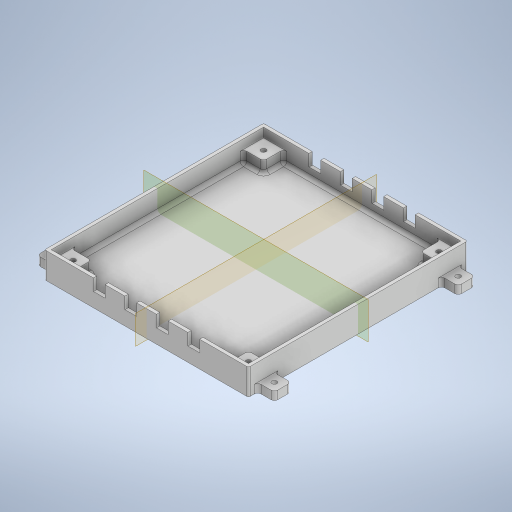
# Autodesk Inventor part: Case
Saved by Autodesk Inventor 2023.5 (Build 275446000, 446)
## iProperties
Created: 2025-10-09
Part Number: Case
Material: Generic
Document SubType Name: Modeling
Designer: Mikke
Density: 1 g/cm^3
Appearance: Default
Author: Mikke
Autodesk Inventor part; units mm, degrees
ref_plane "YZ Plane" through (0, 0, 0) normal (1, 0, 0) x (0, 1, 0)
ref_plane "XZ Plane" through (0, 0, 0) normal (0, 1, 0) x (-1, 0, 0)
ref_plane "XY Plane" through (0, 0, 0) normal (0, 0, 1) x (1, 0, 0)
sketch "Sketch1" plane through (0, 0, 0) normal (0, 1, 0) x (-1, 0, 0)
  line L0 (-61, 65.5) -> (61, 65.5)
  line L1 (61, 65.5) -> (61, -65.5)
  line L2 (61, -65.5) -> (-61, -65.5)
  line L3 (-61, -65.5) -> (-61, 65.5)
  line L4 (-61, 65.5) -> (61, -65.5) construction
  line L5 (61, 65.5) -> (-61, -65.5) construction
  point P0 (0, 0)
  dimension "d0" = 122
  dimension "d1" = 131
  constraints: 12 end point, 2 midpoint, 2 parallel, 1 horizontal, 1 perpendicular
  measures "d0" distance of L1.end L2.end
  measures "d1" distance of L0.end L1.end
extrude "Extrusion1" add sketch "Sketch1" along normal blind 3
sketch "Sketch2" plane through (0, 3, 0) normal (0, 1, 0) x (1, 0, 0)
  line L0 (59, -63.5) -> (-59, -63.5)
  line L1 (-59, -63.5) -> (-59, 63.5)
  line L2 (-59, 63.5) -> (59, 63.5)
  line L3 (59, 63.5) -> (59, -63.5)
  line L4 (59, -63.5) -> (-59, 63.5) construction
  line L5 (-59, -63.5) -> (59, 63.5) construction
  line L6 (-59, -63.5) -> (-53, -63.5)
  line L7 (-53, -63.5) -> (-53, -57.5)
  line L8 (-53, -57.5) -> (-59, -57.5)
  line L9 (-59, -57.5) -> (-59, -63.5)
  line L10 (-59, 63.5) -> (-53, 63.5)
  line L11 (-53, 63.5) -> (-53, 57.5)
  line L12 (-53, 57.5) -> (-59, 57.5)
  line L13 (-59, 57.5) -> (-59, 63.5)
  circle A0 centre (-53, -57.5) radius 1.5
  line L14 (-59, -63.5) -> (-47, -63.5)
  line L15 (-47, -63.5) -> (-47, -51.5)
  line L16 (-47, -51.5) -> (-59, -51.5)
  line L17 (-59, -51.5) -> (-59, -63.5)
  circle A1 centre (-53, 57.5) radius 1.5
  line L18 (-59, 63.5) -> (-47, 63.5)
  line L19 (-47, 63.5) -> (-47, 51.5)
  line L20 (-47, 51.5) -> (-59, 51.5)
  line L21 (-59, 51.5) -> (-59, 63.5)
  line L22 (59, 63.5) -> (53, 63.5)
  line L23 (53, 63.5) -> (53, 57.5)
  line L24 (53, 57.5) -> (59, 57.5)
  line L25 (59, 57.5) -> (59, 63.5)
  line L26 (59, 63.5) -> (47, 63.5)
  line L27 (47, 63.5) -> (47, 51.5)
  line L28 (47, 51.5) -> (59, 51.5)
  line L29 (59, 51.5) -> (59, 63.5)
  circle A2 centre (53, 57.5) radius 1.5
  line L30 (59, -63.5) -> (53, -63.5)
  line L31 (53, -63.5) -> (53, -57.5)
  line L32 (53, -57.5) -> (59, -57.5)
  line L33 (59, -57.5) -> (59, -63.5)
  line L34 (59, -63.5) -> (47, -63.5)
  line L35 (47, -63.5) -> (47, -51.5)
  line L36 (47, -51.5) -> (59, -51.5)
  line L37 (59, -51.5) -> (59, -63.5)
  circle A3 centre (53, -57.5) radius 1.5
  point P0 (0, 0)
  dimension "d4" = 118
  dimension "d5" = 127
  dimension "d6" = 6
  dimension "d7" = 6
  dimension "d8" = 6
  dimension "d9" = 6
  dimension "d11" = 3
  dimension "d12" = 12
  dimension "d13" = 12
  dimension "d14" = 3
  dimension "d15" = 12
  dimension "d16" = 12
  dimension "d17" = 6
  dimension "d18" = 6
  dimension "d19" = 12
  dimension "d20" = 12
  dimension "d21" = 3
  dimension "d22" = 6
  dimension "d23" = 6
  dimension "d24" = 12
  dimension "d25" = 12
  dimension "d26" = 3
  constraints: 76 end point, 18 parallel, 9 horizontal, 9 perpendicular, 4 centre point, 4 coincident, 2 midpoint
  measures "d4" distance of L1.end L2.end
  measures "d5" distance of L0.end L1.end
  measures "d6" distance of L8.end L7.end
  measures "d7" distance of L7.end L6.end
  measures "d8" distance of L11.end L12.end
  measures "d9" distance of L10.end L11.end
  measures "d11" diameter of A0
  measures "d12" distance of L16.end L15.end
  measures "d13" distance of L15.end L14.end
  measures "d14" diameter of A1
  measures "d15" distance of L19.end L20.end
  measures "d16" distance of L18.end L19.end
  measures "d17" distance of L24.end L23.end
  measures "d18" distance of L23.end L22.end
  measures "d19" distance of L28.end L27.end
  measures "d20" distance of L27.end L26.end
  measures "d21" diameter of A2
  measures "d22" distance of L31.end L32.end
  measures "d23" distance of L30.end L31.end
  measures "d24" distance of L35.end L36.end
  measures "d25" distance of L34.end L35.end
  measures "d26" diameter of A3
extrude "Extrusion2" add sketch "Sketch2" along normal blind 7 contours L0 L31 A3 L32 L3 | L0 L35 L36 L3 L32 A3 L31 | A3 L32 L31 | L31 L32 A3 | L0 L7 A0 L8 L1 L16 L15 | L28 L27 L2 L23 A2 L24 L3 | L0 L1 L8 A0 L7 | L24 A2 L23 L2 L3 | A0 L8 L7 | L7 L8 A0 | A2 L23 L24 | L24 L23 A2 | L1 L12 A1 L11 L2 L19 L20 | L1 L2 L11 A1 L12 | A1 L11 L12 | L12 L11 A1
sketch "Sketch3" plane through (0, 3, 0) normal (0, 1, 0) x (1, 0, 0)
  line L0 (-61, 65.5) -> (-61, -65.5) projected
  line L1 (61, 65.5) -> (-61, 65.5) projected
  line L2 (-61, -65.5) -> (61, -65.5)
  line L3 (61, -65.5) -> (61, 65.5)
  line L4 (61, 65.5) -> (-61, 65.5)
  line L5 (-61, 65.5) -> (-61, -65.5)
  line L6 (-59, -63.5) -> (-59, -51.5) projected
  line L7 (59, 63.5) -> (59, 51.5) projected
  line L8 (-59, -63.5) -> (59, -63.5)
  line L9 (59, -63.5) -> (59, 63.5)
  line L10 (59, 63.5) -> (-59, 63.5)
  line L11 (-59, 63.5) -> (-59, -63.5)
  point P0 (0, 0)
  constraints: 16 end point, 4 parallel, 2 horizontal, 2 perpendicular
extrude "Extrusion3" add sketch "Sketch3" along normal blind 12.5
sketch "Sketch5" plane through (47, 3, 63.5) normal (0, 0, -1) x (-1, 0, 0)
  line L0 (-12, 12.5) -> (106, 12.5) projected
  line L1 (0, 7) -> (94, 7)
  line L2 (94, 7) -> (94, 8.5)
  line L3 (94, 8.5) -> (0, 8.5)
  line L4 (0, 8.5) -> (0, 7)
  line L5 (47, 12.5) -> (47, 8.5)
  line L6 (47, 8.5) -> (0, 8.5)
  line L7 (47, 8.5) -> (94, 8.5)
  line L8 (47, 8.5) -> (18.642, 8.5)
  line L9 (47, 8.5) -> (37.575, 8.5)
  line L10 (47, 8.5) -> (56.425, 8.5)
  line L11 (56.425, 8.5) -> (75.283, 8.5)
  line L12 (37.575, 8.5) -> (18.717, 8.5)
  line L13 (18.717, 8.5) -> (18.717, 9)
  line L14 (37.575, 8.5) -> (37.575, 9)
  line L15 (56.425, 8.5) -> (56.425, 9)
  line L16 (75.283, 8.5) -> (75.283, 9)
  line L17 (71.783, 5.5) -> (78.783, 5.5)
  line L18 (78.783, 5.5) -> (78.783, 12.5)
  line L19 (78.783, 12.5) -> (71.783, 12.5)
  line L20 (71.783, 12.5) -> (71.783, 5.5)
  line L21 (71.783, 5.5) -> (78.783, 12.5) construction
  line L22 (78.783, 5.5) -> (71.783, 12.5) construction
  line L23 (52.925, 5.5) -> (59.925, 5.5)
  line L24 (59.925, 5.5) -> (59.925, 12.5)
  line L25 (59.925, 12.5) -> (52.925, 12.5)
  line L26 (52.925, 12.5) -> (52.925, 5.5)
  line L27 (52.925, 5.5) -> (59.925, 12.5) construction
  line L28 (59.925, 5.5) -> (52.925, 12.5) construction
  line L29 (34.075, 5.5) -> (41.075, 5.5)
  line L30 (41.075, 5.5) -> (41.075, 12.5)
  line L31 (41.075, 12.5) -> (34.075, 12.5)
  line L32 (34.075, 12.5) -> (34.075, 5.5)
  line L33 (34.075, 5.5) -> (41.075, 12.5) construction
  line L34 (41.075, 5.5) -> (34.075, 12.5) construction
  line L35 (15.217, 5.5) -> (22.217, 5.5)
  line L36 (22.217, 5.5) -> (22.217, 12.5)
  line L37 (22.217, 12.5) -> (15.217, 12.5)
  line L38 (15.217, 12.5) -> (15.217, 5.5)
  line L39 (15.217, 5.5) -> (22.217, 12.5) construction
  line L40 (22.217, 5.5) -> (15.217, 12.5) construction
  point P0 (47, -3)
  point P1 (47, -3)
  dimension "d31" = 1.5
  dimension "d33" = 9.425
  dimension "d34" = 9.425
  dimension "d35" = 18.858
  dimension "d36" = 18.858
  dimension "d37" = 0.5
  dimension "d38" = 0.5
  dimension "d39" = 0.5
  dimension "d40" = 0.5
  dimension "d41" = 7
  dimension "d42" = 7
  dimension "d43" = 7
  dimension "d44" = 7
  dimension "d45" = 7
  dimension "d46" = 7
  dimension "d47" = 7
  dimension "d48" = 7
  constraints: 80 end point, 10 midpoint, 9 equal length, 8 perpendicular, 5 horizontal, 5 point on line, 3 vertical, 1 coincident
  measures "d31" distance of L1.end L2.end
  measures "d33" distance of L5.end L9.end
  measures "d34" distance of L5.end L10.end
  measures "d35" distance of L10.end L11.end
  measures "d36" distance of L9.end L12.end
  measures "d37" distance of L12.end L13.end
  measures "d38" distance of L9.end L14.end
  measures "d39" distance of L10.end L15.end
  measures "d40" distance of L11.end L16.end
  measures "d41" distance of L19.end L18.end
  measures "d42" distance of L18.end L17.end
  measures "d43" distance of L25.end L24.end
  measures "d44" distance of L24.end L23.end
  measures "d45" distance of L31.end L30.end
  measures "d46" distance of L30.end L29.end
  measures "d47" distance of L37.end L36.end
  measures "d48" distance of L36.end L35.end
extrude "Extrusion4" cut sketch "Sketch5" against normal blind 3 contours L0 L36 L3 L38 | L3 L36 L1 L38 | L0 L30 L3 L32 | L1 L36 L35 L38 | L3 L30 L1 L32 | L1 L30 L29 L32 | L0 L24 L3 L26 | L3 L24 L1 L26 | L1 L24 L23 L26 | L0 L18 L3 L20 | L3 L18 L1 L20 | L1 L18 L17 L20
ref_plane "Work Plane1" through (47, 3, 0) normal (0, 0, -1) x (-1, 0, 0)
mirror "Mirror1" about plane through (47, 3, 0) normal (0, 0, -1) of "Extrusion4"
fillet "Fillet1" radius 2 24 edges at (-47, 3, 57.5) (0, 3, 63.5) (-53, 3, 51.5) (-47, 6.5, 51.5) (-47, 6.5, 63.5) (-59, 6.5, 51.5) (-59, 3, 0) (47, 3, 57.5) (47, 6.5, 51.5) (47, 6.5, 63.5) (53, 3, 51.5) (59, 3, 0) (59, 6.5, 51.5) (53, 3, -51.5) (59, 6.5, -51.5) (47, 6.5, -51.5) (47, 3, -57.5) (47, 6.5, -63.5) (0, 3, -63.5) (-59, 6.5, -51.5) (-53, 3, -51.5) (-47, 6.5, -51.5) (-47, 3, -57.5) (-47, 6.5, -63.5)
fillet "Fillet2" radius 1 4 edges at (-61, 7.75, -65.5) (61, 7.75, -65.5) (61, 7.75, 65.5) (-61, 7.75, 65.5)
sketch "Sketch6" plane through (0, 10, 0) normal (0, 1, 0) x (1, 0, 0)
  line L0 (-59, -63.5) -> (-45, -63.5) projected
  line L1 (-59, -63.5) -> (-47, -63.5)
  line L2 (-47, -63.5) -> (-47, -51.5)
  line L3 (-47, -51.5) -> (-59, -51.5)
  line L4 (-59, -51.5) -> (-59, -63.5)
  line L5 (-59, -63.5) -> (-52.5, -63.5)
  line L6 (-52.5, -63.5) -> (-52.5, -57)
  line L7 (-52.5, -57) -> (-59, -57)
  line L8 (-59, -57) -> (-59, -63.5)
  circle A0 centre (-52.5, -57) radius 1.5
  point P0 (0, 0)
  dimension "d53" = 12
  dimension "d54" = 12
  dimension "d55" = 6.5
  dimension "d56" = 6.5
  dimension "d57" = 3
  constraints: 16 end point, 4 parallel, 2 horizontal, 2 perpendicular, 1 centre point, 1 coincident
  measures "d53" distance of L3.end L2.end
  measures "d54" distance of L2.end L1.end
  measures "d55" distance of L7.end L6.end
  measures "d56" distance of L6.end L5.end
  measures "d57" diameter of A0
extrude "Extrusion5" cut sketch "Sketch6" against normal blind 7 contours A0 L7 L6 | L6 L7 A0
ref_plane "Work Plane2" through (0, 10, -63.5) normal (1, 0, 0) x (0, 0, -1)
mirror "Mirror2" about plane through (0, 10, -63.5) normal (1, 0, 0) of "Extrusion5"
mirror "Mirror3" about plane through (47, 3, 0) normal (0, 0, -1) of "Extrusion5", "Mirror2"
sketch "Sketch7" plane through (0, 0, 0) normal (0, -1, 0) x (1, 0, 0)
  line L0 (-61, -64.5) -> (-61, 64.5) projected
  line L1 (-61, 60) -> (-69, 60)
  line L2 (-71, 58) -> (-71, 52)
  line L3 (-69, 50) -> (-61, 50)
  line L4 (-61, 50) -> (-61, 60)
  circle A0 centre (-66, 55) radius 1.5
  arc A1 (-69, 60) -> (-71, 58) centre (-69, 58) ccw
  arc A2 (-71, 52) -> (-69, 50) centre (-69, 52) ccw
  point P0 (0, 0)
  point P1 (-71, 50)
  point P2 (-71, 60)
  dimension "d60" = 10
  dimension "d61" = 10
  dimension "d62" = 3
  dimension "d63" = 2
  constraints: 8 end point, 5 point on line, 4 point on circle, 4 tangent, 3 centre point, 2 parallel, 1 coincident, 1 equal radius, 1 horizontal, 1 perpendicular
  measures "d60" distance of L3.end point (-71, 50)
  measures "d61" distance of point (-71, 50) point (-71, 60)
  measures "d62" diameter of A0
  measures "d63" radius of A1
extrude "Extrusion6" add sketch "Sketch7" against normal blind 5
mirror "Mirror4" about plane through (0, 10, -63.5) normal (1, 0, 0) of "Extrusion6"
mirror "Mirror5" about plane through (47, 3, 0) normal (0, 0, -1) of "Extrusion6", "Mirror4"
fillet "Fillet3" radius 2 8 edges at (-61, 2.5, 60) (-61, 2.5, 50) (-61, 2.5, -50) (-61, 2.5, -60) (61, 2.5, 60) (61, 2.5, -50) (61, 2.5, -60) (61, 2.5, 50)
body "Solid1"
